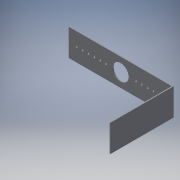
# Autodesk Inventor part: Gimbal UP DoWN
Saved by Autodesk Inventor 2016 (Build 200138000, 138)
## iProperties
Created: 2016-02-12
Part Number: Gimbal UP DoWN
Material: Generic
Document SubType Name: Modeling
Designer: RoksBot
Density: 1 g/cm^3
Appearance: Default
Author: RoksBot
Autodesk Inventor part; units mm, degrees
ref_plane "YZ Plane" through (0, 0, 0) normal (1, 0, 0) x (0, 1, 0)
ref_plane "XZ Plane" through (0, 0, 0) normal (0, 1, 0) x (-1, 0, 0)
ref_plane "XY Plane" through (0, 0, 0) normal (0, 0, 1) x (1, 0, 0)
sketch "Sketch1" plane through (0, 0, 0) normal (0, 0, 1) x (1, 0, 0)
  line L0 (12.283962, 2.6543) -> (-0.123022, 1.811929)
  circle A0 centre (19.303998, 0) radius 0.3429
  circle A1 centre (21.208998, 0) radius 0.3429
  circle A2 centre (23.113998, 0) radius 0.3429
  circle A3 centre (25.018998, 0) radius 0.3429
  circle A4 centre (26.923998, 0) radius 0.3429
  circle A5 centre (28.828998, 0) radius 0.3429
  circle A6 centre (9.524998, 0) radius 0.3429
  circle A7 centre (7.619998, 0) radius 0.3429
  circle A8 centre (5.714998, 0) radius 0.3429
  circle A9 centre (3.809998, 0) radius 0.3429
  circle A10 centre (1.904998, 0) radius 0.3429
  circle A11 centre (-0.000002, 0) radius 0.3429
  circle A12 centre (14.414498, 0) radius 2.6162
  arc A13 (-0.123022, 1.811929) -> (-0.123022, -1.811929) centre (-0.000002, 0) ccw
  line L1 (-0.123022, -1.811929) -> (12.283962, -2.6543)
  arc A14 (12.283962, -2.6543) -> (16.545035, -2.6543) centre (14.414498, 0) ccw
  line L2 (16.545035, -2.6543) -> (28.952019, -1.811929)
  arc A15 (28.952019, -1.811929) -> (28.952019, 1.811929) centre (28.828998, 0) ccw
  line L3 (28.952019, 1.811929) -> (16.545035, 2.6543)
  arc A16 (16.545035, 2.6543) -> (12.283962, 2.6543) centre (14.414498, 0) ccw
  line L4 (12.283962, 2.6543) -> (-0.123022, 1.811929)
  line L5 (33.756598, -5.02492) -> (-4.927602, -5.02492)
  line L6 (-4.927602, -5.02492) -> (-4.927602, 5.02492)
  line L7 (-4.927602, 5.02492) -> (33.756598, 5.02492)
  line L8 (33.756598, 5.02492) -> (33.756598, -5.02492)
  line L9 (33.756598, -5.02492) -> (-4.927602, 5.02492) construction
  line L10 (-4.927602, -5.02492) -> (33.756598, 5.02492) construction
  point P0 (0, 0)
  constraints: 12 end point, 2 midpoint, 2 parallel, 1 horizontal, 1 perpendicular
extrude "Extrusion1" add sketch "Sketch1" along normal blind 2.54 contours A16 L3 A15 L2 A14 L1 A13 L0 | L5 L6 L7 L8
fillet "Fillet1" radius 3.175 2 edges at (-4.9276, 5.0249, 1.27) (-4.9276, -5.0249, 1.27)
sketch "Sketch3" plane through (0, 0, 0) normal (0, 0, -1) x (-1, 0, 0)
  line L0 (-65.150998, -16.63483) -> (-48.590198, -16.63483)
  line L1 (-48.590198, 5.99657) -> (-65.150998, 5.99657)
  line L2 (-33.756598, -5.02492) -> (1.752602, -5.02492)
  line L3 (1.752602, 5.02492) -> (-33.756598, 5.02492)
  line L4 (-33.756598, 5.02492) -> (-33.756598, -5.02492)
  line L5 (-54.940198, -21.62593) -> (-42.062398, -21.62593)
  line L6 (-42.062398, -21.62593) -> (-42.062398, 10.98767)
  line L7 (-42.062398, 10.98767) -> (-54.940198, 10.98767)
  line L8 (-54.940198, 10.98767) -> (-54.940198, -21.62593)
  line L9 (-48.590198, -21.11793) -> (-48.590198, -16.12683)
  line L10 (-42.062398, -10.75473) -> (-42.062398, -16.12683)
  line L11 (-33.756598, 5.02492) -> (1.752602, 5.02492)
  arc A0 (-33.756598, -5.02492) -> (-42.062398, -21.62593) centre (-21.319073, -21.62593) ccw
  arc A1 (-42.062398, 10.98767) -> (-33.756598, 5.02492) centre (-35.769163, 10.98767) ccw
  line L12 (-48.590198, 10.98767) -> (-46.558198, 10.98767)
  line L13 (-46.558198, -21.62593) -> (-48.590198, -21.62593)
  point P0 (0, 0)
  dimension "d8" = 6.35
  constraints: 8 end point, 4 point on circle, 3 point on line, 2 centre point, 2 parallel, 2 tangent, 1 horizontal, 1 perpendicular
  measures "d8" distance between parallel lines of L9 L8
extrude "Extrusion3" add sketch "Sketch3" against normal up to surface (2.54 mm away)
fillet "Fillet2" radius 3.175 4 edges at (33.7566, -5.0249, 1.27) (33.7566, 5.0249, 1.27) (42.0624, 10.9877, 1.27) (42.0624, -21.6259, 1.27)
fillet "Fillet3" radius 1.27 13 edges at (33.7401, -5.2179, 0) (15.4487, -5.0249, 0) (-3.9977, -4.095, 0) (-4.9276, 0, 0) (-3.9977, 4.095, 0) (15.7684, 5.0249, 0) (33.7089, 4.9971, 0) (38.686, 5.4112, 0) (42.8589, 10.407, 0) (49.8147, 10.9877, 0) (42.935, -20.8404, 0) (49.983, -21.6259, 0) (39.5083, -11.6541, 0)
fillet "Fillet4" radius 1.27 5 edges at (54.9402, -21.254, 0.372) (54.9402, -5.3191, 0) (54.9402, 10.6157, 0.372) (54.9402, 10.9877, 1.905) (54.9402, -21.6259, 1.905)
sketch "Sketch4" plane through (0, 0, 2.54) normal (0, 0, 1) x (1, 0, 0)
  line L0 (48.590198, 10.47967) -> (48.590198, 5.48857)
  line L1 (65.150998, 5.99657) -> (48.590198, 5.99657)
  line L2 (48.590198, -16.12683) -> (48.590198, -21.11793)
  line L3 (48.590198, -16.63483) -> (65.150998, -16.63483)
  line L4 (48.590198, 6.15532) -> (54.940198, 6.15532)
  line L5 (48.590198, 9.71767) -> (48.590198, 6.15532)
  line L6 (54.940198, -19.33358) -> (48.590198, -19.33358)
  line L7 (48.590198, -19.33358) -> (48.590198, -16.79358)
  line L8 (48.590198, -16.79358) -> (54.940198, -16.79358)
  line L9 (54.940198, -16.79358) -> (54.940198, -19.33358)
  line L10 (48.590198, -16.79358) -> (49.860198, -16.79358)
  line L11 (49.860198, -16.79358) -> (49.860198, -21.62593)
  line L12 (49.860198, -21.62593) -> (48.590198, -21.62593)
  line L13 (48.590198, -21.62593) -> (48.590198, -16.79358)
  line L14 (48.590198, 6.15532) -> (49.860198, 6.15532)
  line L15 (49.860198, 6.15532) -> (49.860198, 10.98767)
  line L16 (49.860198, 10.98767) -> (48.590198, 10.98767)
  line L17 (48.590198, 10.98767) -> (48.590198, 6.15532)
  line L18 (44.689189, 10.98767) -> (53.670198, 10.98767)
  line L19 (53.670198, -21.62593) -> (45.025732, -21.62593)
  line L20 (48.590198, 6.15532) -> (54.940198, 6.15532)
  line L21 (54.940198, 6.15532) -> (54.940198, 8.69532)
  line L22 (54.940198, 8.69532) -> (48.590198, 8.69532)
  line L23 (48.590198, 8.69532) -> (48.590198, 6.15532)
  line L24 (54.940198, 9.71767) -> (54.940198, -20.35593)
  point P0 (0, 0)
  dimension "d14" = 0.15875
  dimension "d15" = 0.15875
  dimension "d18" = 1.27
  dimension "d25" = 2.54
  dimension "d26" = 2.54
  constraints: 36 end point, 7 parallel, 7 point on line, 5 horizontal, 4 perpendicular, 2 vertical alignment
  measures "d14" distance between parallel lines of L1 L4
  measures "d15" distance between parallel lines of L3 L8
  measures "d18" distance between parallel lines of L0 L15
  measures "d25" distance between parallel lines of L8 L6
  measures "d26" distance between parallel lines of L4 L22
ref_plane "Work Plane1" through (42.062398, -21.11793, 17.4752) normal (0, 0, 1) x (1, 0, 0)
extrude "Extrusion4" add sketch "Sketch4" along normal up to surface (14.9352 mm away) contours L17 L16 L15 L22 L0 | L22 L15 L4 L0 | L22 L21 L4 L15 | L8 L11 L6 L2 | L6 L11 L12 L13 L2 | L8 L9 L6 L11
fillet "Fillet5" radius 0.508 3 edges at (52.4002, -19.3336, 2.54) (49.8602, -20.4798, 2.54) (49.8602, 9.8415, 2.54)
fillet "Fillet6" radius 3.175 4 edges at (54.9402, -18.0636, 17.4752) (54.9402, 7.4253, 17.4752) (49.2252, 10.9877, 17.4752) (49.2252, -21.6259, 17.4752)
sketch "Sketch5" plane through (54.940198, -20.35593, 1.27) normal (1, 0, 0) x (0, 0, -1)
  line L0 (-4.445, 25.8445) -> (-4.445, 4.2291)
  line L1 (-1.27, 14.582398) -> (-1.27, 1.48354)
  line L2 (-1.27, 26.51125) -> (-16.2052, 26.51125)
  line L3 (-1.27, 1.48354) -> (-4.445, 1.48354)
  line L4 (-4.445, 1.48354) -> (-4.445, 26.51125)
  line L5 (-4.445, 26.51125) -> (-1.27, 26.51125)
  line L6 (-1.27, 26.51125) -> (-1.27, 1.48354)
  point P0 (1.27, 20.35593)
  point P1 (-16.2052, 24.37765)
  constraints: 8 end point, 2 parallel, 1 horizontal, 1 perpendicular, 1 point on line, 2 other
ref_plane "Work Plane2" through (42.062398, -16.63483, 5.715) normal (-1, 0, 0) x (0, 0, 1)
extrude "Extrusion5" add sketch "Sketch5" against normal up to surface (12.8778 mm away)
fillet "Fillet7" radius 3.175 1 edges at (42.0624, -6.3585, 2.54)
fillet "Fillet8" radius 1.27 4 edges at (45.2345, -18.8724, 2.54) (44.1954, 6.1553, 2.54) (48.5902, 8.5715, 2.54) (48.5902, -20.2492, 2.54)
sketch "Sketch6" plane through (48.590198, -16.79358, 5.715) normal (-1, 0, 0) x (0, 0, 1)
  arc A0 (5.2705, 26.120191) -> (6.4897, 26.120191) centre (5.8801, 25.35555) ccw
  arc A1 (6.4897, -3.171291) -> (5.2705, -3.171291) centre (5.8801, -2.40665) ccw
  circle A2 centre (5.8801, 25.35555) radius 0.762
  circle A3 centre (5.8801, -2.40665) radius 0.762
  point P0 (-5.715, 16.79358)
  dimension "d27" = 1.524
  constraints: 2 centre point, 2 coincident, 1 equal radius
  measures "d27" diameter of A2
extrude "Extrusion6" cut sketch "Sketch6" against normal through all
equation "\"d15\" = d14"
equation "\"d26\" = d25"
body "Solid1"
